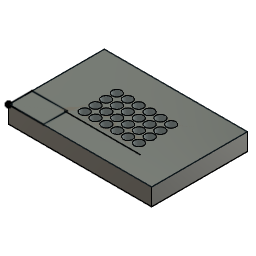
PDT LED Original Array Case Cover v6 (Autodesk Fusion 360 design; units mm, degrees)
Autodesk Fusion 360 part; units mm, degrees
sketch "Sketch1" plane through (0, 0, 0) normal (0, 1, 0) x (1, 0, 0)
  line L0 (0, 0) -> (250, 0)
  line L1 (250, 0) -> (250, -167.253)
  line L2 (250, -167.253) -> (0, -167.253)
  line L3 (0, -167.253) -> (0, 0)
  dimension "d1" = 167.253
  dimension "d2" = 250
  constraint horizontal L0
  constraint vertical L1
  constraint horizontal L2
  constraint vertical L3
  constraint coincident L0.start L3.end
  measures "d1" distance of L0.start L2.end
  measures "d2" distance of L0.start L0.end
extrude "Extrude1" add sketch "Sketch1" along normal blind 30 makes body 1
sketch "Sketch2" plane through (0, 0, 0) normal (0, 1, 0) x (1, 0, 0)
  line L0 (0, 25) -> (127.8, 25)
  line L1 (127.8, 25) -> (127.8, 110.2)
  line L2 (127.8, 110.2) -> (0, 110.2)
  line L3 (0, 110.2) -> (0, 25)
  dimension "d5" = 85.2
  dimension "d6" = 127.8
  constraint horizontal L0
  constraint vertical L1
  constraint horizontal L2
  constraint vertical L3
  measures "d5" distance of L0.start L2.end
  measures "d6" distance of L0.start L0.end
extrude "Extrude2" add sketch "Sketch2" along normal blind 15 separate body makes body 2
sketch "Sketch3" plane through (0, 15, 0) normal (0, 1, 0) x (-1, 0, 0)
  line L0 (0, -110.2) -> (0, -25)
  line L1 (0, -25) -> (-127.8, -25)
  line L2 (-127.8, -25) -> (-127.8, -110.2)
  line L3 (-127.8, -110.2) -> (0, -110.2)
  line L4 (0, -110.2) -> (-16.5, -110.2)
  line L5 (-16.5, -110.2) -> (-16.5, -124.6)
  line L6 (-16.5, -124.6) -> (0, -124.6)
  line L7 (0, -124.6) -> (0, -110.2)
  dimension "d9" = 14.4
  dimension "d10" = 16.5
  constraint horizontal L4
  constraint vertical L5
  constraint horizontal L6
  constraint vertical L7
  constraint coincident L0.start L3.end
  measures "d9" distance of L0.start L6.end
  measures "d10" distance of L0.start L4.end
move_body "Move1" bodies 2 to x (1, 0, 0) y (0, 1, 0) z (0, 0, 1) at (0, 0, -14.638)
hole "Hole1" at (16.5, 15, -110.2) direction (0, -1, 0) diameter 16.3 depth 15 tip angle 118 bodies 2
sketch "Sketch4" plane through (0, 15, 0) normal (0, 1, 0) x (-1, 0, 0)
  circle A0 centre (-16.5, -110.2) radius 8.15
  line L0 (0, -124.838) -> (0, -39.638)
  line L1 (0, -39.638) -> (-127.8, -39.638)
  line L2 (-127.8, -39.638) -> (-127.8, -124.838)
  line L3 (-127.8, -124.838) -> (0, -124.838)
  line L4 (0, -39.638) -> (-16.5, -39.638)
  line L5 (-16.5, -39.638) -> (-16.5, -54.038)
  line L6 (-16.5, -54.038) -> (0, -54.038)
  line L7 (0, -54.038) -> (0, -39.638)
  dimension "d14" = 16.5
  dimension "d15" = 14.4
  constraint horizontal L4
  constraint vertical L5
  constraint horizontal L6
  constraint vertical L7
  constraint coincident L0.end L1.start
  measures "d14" distance of L0.end L4.end
  measures "d15" distance of L0.end L6.end
hole "Hole2" at (16.5, 15, -54.038) direction (0, -1, 0) diameter 16.3 depth 15 tip angle 118 bodies 2
sketch "Sketch5" plane through (0, 15, 0) normal (0, 1, 0) x (-1, 0, 0)
  circle A0 centre (-16.5, -54.038) radius 8.15
  circle A1 centre (-16.5, -110.2) radius 8.15
  line L0 (0, -124.838) -> (0, -39.638)
  line L1 (0, -39.638) -> (-127.8, -39.638)
  line L2 (-127.8, -39.638) -> (-127.8, -124.838)
  line L3 (-127.8, -124.838) -> (0, -124.838)
  line L4 (0, -39.638) -> (-16.5, -39.638)
  line L5 (-16.5, -39.638) -> (-16.5, -72.938)
  line L6 (-16.5, -72.938) -> (0, -72.938)
  line L7 (0, -72.938) -> (0, -39.638)
  dimension "d19" = 33.3
  dimension "d20" = 16.5
  constraint horizontal L4
  constraint vertical L5
  constraint horizontal L6
  constraint vertical L7
  constraint coincident L0.end L1.start
  measures "d19" distance of L0.end L6.end
  measures "d20" distance of L0.end L4.end
hole "Hole3" at (16.5, 15, -72.938) direction (0, -1, 0) diameter 16.3 depth 15 tip angle 118 bodies 2
sketch "Sketch6" plane through (0, 15, 0) normal (0, 1, 0) x (-1, 0, 0)
  circle A0 centre (-16.5, -72.938) radius 8.15
  circle A1 centre (-16.5, -54.038) radius 8.15
  circle A2 centre (-16.5, -110.2) radius 8.15
  line L0 (0, -124.838) -> (0, -39.638)
  line L1 (0, -39.638) -> (-127.8, -39.638)
  line L2 (-127.8, -39.638) -> (-127.8, -124.838)
  line L3 (-127.8, -124.838) -> (0, -124.838)
  line L4 (0, -124.838) -> (-16.5, -124.838)
  line L5 (-16.5, -124.838) -> (-16.5, -91.538)
  line L6 (-16.5, -91.538) -> (0, -91.538)
  line L7 (0, -91.538) -> (0, -124.838)
  dimension "d24" = 33.3
  dimension "d25" = 16.5
  constraint horizontal L4
  constraint vertical L5
  constraint horizontal L6
  constraint vertical L7
  constraint coincident L0.start L3.end
  measures "d24" distance of L0.start L6.end
  measures "d25" distance of L0.start L4.end
hole "Hole4" at (16.5, 15, -91.538) direction (0, -1, 0) diameter 16.3 depth 15 tip angle 118 bodies 2
sketch "Sketch7" plane through (0, 0, -39.638) normal (0, 0, 1) x (1, 0, 0)
  line L0 (0, 0) -> (127.8, 0)
  line L1 (127.8, 0) -> (127.8, 15)
  line L2 (127.8, 15) -> (0, 15)
  line L3 (0, 15) -> (0, 0)
sketch "Sketch8" plane through (0, 15, 0) normal (0, 1, 0) x (-1, 0, 0)
  circle A0 centre (-16.5, -91.538) radius 8.15
  circle A1 centre (-16.5, -72.938) radius 8.15
  circle A2 centre (-16.5, -54.038) radius 8.15
  circle A3 centre (-16.5, -110.2) radius 8.15
  line L0 (0, -124.838) -> (0, -39.638)
  line L1 (0, -39.638) -> (-127.8, -39.638)
  line L2 (-127.8, -39.638) -> (-127.8, -124.838)
  line L3 (-127.8, -124.838) -> (0, -124.838)
  line L4 (0, -39.638) -> (-35.4, -39.638)
  line L5 (-35.4, -39.638) -> (-35.4, -54.038)
  line L6 (-35.4, -54.038) -> (0, -54.038)
  line L7 (0, -54.038) -> (0, -39.638)
  dimension "d29" = 35.4
  dimension "d30" = 14.4
  constraint horizontal L4
  constraint vertical L5
  constraint horizontal L6
  constraint vertical L7
  constraint coincident L0.end L1.start
  measures "d29" distance of L0.end L4.end
  measures "d30" distance of L0.end L6.end
hole "Hole5" at (35.4, 15, -54.038) direction (0, -1, 0) diameter 16.3 depth 15 tip angle 118 bodies 2
sketch "Sketch9" plane through (0, 15, 0) normal (0, 1, 0) x (-1, 0, 0)
  circle A0 centre (-35.4, -54.038) radius 8.15
  circle A1 centre (-16.5, -91.538) radius 8.15
  circle A2 centre (-16.5, -72.938) radius 8.15
  circle A3 centre (-16.5, -54.038) radius 8.15
  circle A4 centre (-16.5, -110.2) radius 8.15
  line L0 (0, -124.838) -> (0, -39.638)
  line L1 (0, -39.638) -> (-127.8, -39.638)
  line L2 (-127.8, -39.638) -> (-127.8, -124.838)
  line L3 (-127.8, -124.838) -> (0, -124.838)
  line L4 (0, -39.638) -> (-35.4, -39.638)
  line L5 (-35.4, -39.638) -> (-35.4, -72.938)
  line L6 (-35.4, -72.938) -> (0, -72.938)
  line L7 (0, -72.938) -> (0, -39.638)
  dimension "d34" = 33.3
  dimension "d35" = 35.4
  constraint horizontal L4
  constraint vertical L5
  constraint horizontal L6
  constraint vertical L7
  constraint coincident L0.end L1.start
  measures "d34" distance of L0.end L6.end
  measures "d35" distance of L0.end L4.end
hole "Hole6" at (35.4, 15, -72.938) direction (0, -1, 0) diameter 16.3 depth 15 tip angle 118 bodies 2
sketch "Sketch10" plane through (0, 15, 0) normal (0, 1, 0) x (-1, 0, 0)
  circle A0 centre (-35.4, -72.938) radius 8.15
  circle A1 centre (-35.4, -54.038) radius 8.15
  circle A2 centre (-16.5, -91.538) radius 8.15
  circle A3 centre (-16.5, -72.938) radius 8.15
  circle A4 centre (-16.5, -54.038) radius 8.15
  circle A5 centre (-16.5, -110.2) radius 8.15
  line L0 (0, -124.838) -> (0, -39.638)
  line L1 (0, -39.638) -> (-127.8, -39.638)
  line L2 (-127.8, -39.638) -> (-127.8, -124.838)
  line L3 (-127.8, -124.838) -> (0, -124.838)
  line L4 (0, -124.838) -> (-35.4, -124.838)
  line L5 (-35.4, -124.838) -> (-35.4, -91.538)
  line L6 (-35.4, -91.538) -> (0, -91.538)
  line L7 (0, -91.538) -> (0, -124.838)
  dimension "d39" = 33.3
  dimension "d40" = 35.4
  constraint horizontal L4
  constraint vertical L5
  constraint horizontal L6
  constraint vertical L7
  constraint coincident L0.start L3.end
  measures "d39" distance of L0.start L6.end
  measures "d40" distance of L0.start L4.end
hole "Hole7" at (35.4, 15, -91.538) direction (0, -1, 0) diameter 16.3 depth 15 tip angle 118 bodies 2
sketch "Sketch11" plane through (0, 15, 0) normal (0, 1, 0) x (-1, 0, 0)
  circle A0 centre (-35.4, -91.538) radius 8.15
  circle A1 centre (-35.4, -72.938) radius 8.15
  circle A2 centre (-35.4, -54.038) radius 8.15
  circle A3 centre (-16.5, -91.538) radius 8.15
  circle A4 centre (-16.5, -72.938) radius 8.15
  circle A5 centre (-16.5, -54.038) radius 8.15
  circle A6 centre (-16.5, -110.2) radius 8.15
  line L0 (0, -124.838) -> (0, -39.638)
  line L1 (0, -39.638) -> (-127.8, -39.638)
  line L2 (-127.8, -39.638) -> (-127.8, -124.838)
  line L3 (-127.8, -124.838) -> (0, -124.838)
  line L4 (0, -124.838) -> (-35.4, -124.838)
  line L5 (-35.4, -124.838) -> (-35.4, -110.438)
  line L6 (-35.4, -110.438) -> (0, -110.438)
  line L7 (0, -110.438) -> (0, -124.838)
  dimension "d44" = 35.4
  dimension "d45" = 14.4
  constraint horizontal L4
  constraint vertical L5
  constraint horizontal L6
  constraint vertical L7
  constraint coincident L0.start L3.end
  measures "d44" distance of L0.start L4.end
  measures "d45" distance of L0.start L6.end
hole "Hole8" at (35.4, 15, -110.438) direction (0, -1, 0) diameter 16.3 depth 15 tip angle 118 bodies 2
sketch "Sketch12" plane through (0, 15, 0) normal (0, 1, 0) x (-1, 0, 0)
  circle A0 centre (-35.4, -110.438) radius 8.15
  circle A1 centre (-35.4, -91.538) radius 8.15
  circle A2 centre (-35.4, -72.938) radius 8.15
  circle A3 centre (-35.4, -54.038) radius 8.15
  circle A4 centre (-16.5, -91.538) radius 8.15
  circle A5 centre (-16.5, -72.938) radius 8.15
  circle A6 centre (-16.5, -54.038) radius 8.15
  circle A7 centre (-16.5, -110.2) radius 8.15
  line L0 (0, -124.838) -> (0, -39.638)
  line L1 (0, -39.638) -> (-127.8, -39.638)
  line L2 (-127.8, -39.638) -> (-127.8, -124.838)
  line L3 (-127.8, -124.838) -> (0, -124.838)
  line L4 (0, -124.838) -> (-54.3, -124.838)
  line L5 (-54.3, -124.838) -> (-54.3, -110.438)
  line L6 (-54.3, -110.438) -> (0, -110.438)
  line L7 (0, -110.438) -> (0, -124.838)
  dimension "d49" = 54.3
  constraint horizontal L4
  constraint vertical L5
  constraint horizontal L6
  constraint vertical L7
  constraint coincident L0.start L3.end
  measures "d49" distance of L0.start L4.end
hole "Hole9" at (54.3, 15, -110.438) direction (0, -1, 0) diameter 16.3 depth 15 tip angle 118 bodies 2
sketch "Sketch13" plane through (0, 15, 0) normal (0, 1, 0) x (-1, 0, 0)
  circle A0 centre (-54.3, -110.438) radius 8.15
  circle A1 centre (-35.4, -110.438) radius 8.15
  circle A2 centre (-35.4, -91.538) radius 8.15
  circle A3 centre (-35.4, -72.938) radius 8.15
  circle A4 centre (-35.4, -54.038) radius 8.15
  circle A5 centre (-16.5, -91.538) radius 8.15
  circle A6 centre (-16.5, -72.938) radius 8.15
  circle A7 centre (-16.5, -54.038) radius 8.15
  circle A8 centre (-16.5, -110.2) radius 8.15
  line L0 (0, -124.838) -> (0, -39.638)
  line L1 (0, -39.638) -> (-127.8, -39.638)
  line L2 (-127.8, -39.638) -> (-127.8, -124.838)
  line L3 (-127.8, -124.838) -> (0, -124.838)
  line L4 (0, -124.838) -> (-54.3, -124.838)
  line L5 (-54.3, -124.838) -> (-54.3, -91.538)
  line L6 (-54.3, -91.538) -> (0, -91.538)
  line L7 (0, -91.538) -> (0, -124.838)
  dimension "d53" = 54.3
  dimension "d54" = 33.3
  constraint horizontal L4
  constraint vertical L5
  constraint horizontal L6
  constraint vertical L7
  constraint coincident L0.start L3.end
  measures "d53" distance of L0.start L4.end
  measures "d54" distance of L0.start L6.end
hole "Hole10" at (54.3, 15, -91.538) direction (0, -1, 0) diameter 16.3 depth 15 tip angle 118 bodies 2
sketch "Sketch14" plane through (0, 15, 0) normal (0, 1, 0) x (-1, 0, 0)
  circle A0 centre (-54.3, -91.538) radius 8.15
  circle A1 centre (-54.3, -110.438) radius 8.15
  circle A2 centre (-35.4, -110.438) radius 8.15
  circle A3 centre (-35.4, -91.538) radius 8.15
  circle A4 centre (-35.4, -72.938) radius 8.15
  circle A5 centre (-35.4, -54.038) radius 8.15
  circle A6 centre (-16.5, -91.538) radius 8.15
  circle A7 centre (-16.5, -72.938) radius 8.15
  circle A8 centre (-16.5, -54.038) radius 8.15
  circle A9 centre (-16.5, -110.2) radius 8.15
  line L0 (0, -124.838) -> (0, -39.638)
  line L1 (0, -39.638) -> (-127.8, -39.638)
  line L2 (-127.8, -39.638) -> (-127.8, -124.838)
  line L3 (-127.8, -124.838) -> (0, -124.838)
  line L4 (0, -39.638) -> (-54.3, -39.638)
  line L5 (-54.3, -39.638) -> (-54.3, -72.938)
  line L6 (-54.3, -72.938) -> (0, -72.938)
  line L7 (0, -72.938) -> (0, -39.638)
  dimension "d58" = 54.3
  dimension "d59" = 33.3
  constraint horizontal L4
  constraint vertical L5
  constraint horizontal L6
  constraint vertical L7
  constraint coincident L0.end L1.start
  measures "d58" distance of L0.end L4.end
  measures "d59" distance of L0.end L6.end
hole "Hole11" at (54.3, 15, -72.938) direction (0, -1, 0) diameter 16.3 depth 15 tip angle 118 bodies 2
sketch "Sketch15" plane through (0, 15, 0) normal (0, 1, 0) x (-1, 0, 0)
  circle A0 centre (-54.3, -72.938) radius 8.15
  circle A1 centre (-54.3, -91.538) radius 8.15
  circle A2 centre (-54.3, -110.438) radius 8.15
  circle A3 centre (-35.4, -110.438) radius 8.15
  circle A4 centre (-35.4, -91.538) radius 8.15
  circle A5 centre (-35.4, -72.938) radius 8.15
  circle A6 centre (-35.4, -54.038) radius 8.15
  circle A7 centre (-16.5, -91.538) radius 8.15
  circle A8 centre (-16.5, -72.938) radius 8.15
  circle A9 centre (-16.5, -54.038) radius 8.15
  circle A10 centre (-16.5, -110.2) radius 8.15
  line L0 (0, -124.838) -> (0, -39.638)
  line L1 (0, -39.638) -> (-127.8, -39.638)
  line L2 (-127.8, -39.638) -> (-127.8, -124.838)
  line L3 (-127.8, -124.838) -> (0, -124.838)
  line L4 (0, -39.638) -> (-54.3, -39.638)
  line L5 (-54.3, -39.638) -> (-54.3, -54.038)
  line L6 (-54.3, -54.038) -> (0, -54.038)
  line L7 (0, -54.038) -> (0, -39.638)
  dimension "d63" = 54.3
  dimension "d64" = 14.4
  constraint horizontal L4
  constraint vertical L5
  constraint horizontal L6
  constraint vertical L7
  constraint coincident L0.end L1.start
  measures "d63" distance of L0.end L4.end
  measures "d64" distance of L0.end L6.end
hole "Hole12" at (54.3, 15, -54.038) direction (0, -1, 0) diameter 16.3 depth 15 tip angle 118 bodies 2
sketch "Sketch16" plane through (0, 15, 0) normal (0, 1, 0) x (-1, 0, 0)
  circle A0 centre (-54.3, -54.038) radius 8.15
  circle A1 centre (-54.3, -72.938) radius 8.15
  circle A2 centre (-54.3, -91.538) radius 8.15
  circle A3 centre (-54.3, -110.438) radius 8.15
  circle A4 centre (-35.4, -110.438) radius 8.15
  circle A5 centre (-35.4, -91.538) radius 8.15
  circle A6 centre (-35.4, -72.938) radius 8.15
  circle A7 centre (-35.4, -54.038) radius 8.15
  circle A8 centre (-16.5, -91.538) radius 8.15
  circle A9 centre (-16.5, -72.938) radius 8.15
  circle A10 centre (-16.5, -54.038) radius 8.15
  circle A11 centre (-16.5, -110.2) radius 8.15
  line L0 (0, -124.838) -> (0, -39.638)
  line L1 (0, -39.638) -> (-127.8, -39.638)
  line L2 (-127.8, -39.638) -> (-127.8, -124.838)
  line L3 (-127.8, -124.838) -> (0, -124.838)
  line L4 (-127.8, -124.838) -> (-73.5, -124.838)
  line L5 (-73.5, -124.838) -> (-73.5, -110.438)
  line L6 (-73.5, -110.438) -> (-127.8, -110.438)
  line L7 (-127.8, -110.438) -> (-127.8, -124.838)
  dimension "d68" = 54.3
  dimension "d69" = 14.4
  constraint horizontal L4
  constraint vertical L5
  constraint horizontal L6
  constraint vertical L7
  constraint coincident L2.end L3.start
  measures "d68" distance of L2.end L4.end
  measures "d69" distance of L2.end L6.end
hole "Hole13" at (73.5, 15, -110.438) direction (0, -1, 0) diameter 16.3 depth 15 tip angle 118 bodies 2
sketch "Sketch17" plane through (0, 15, 0) normal (0, 1, 0) x (-1, 0, 0)
  circle A0 centre (-73.5, -110.438) radius 8.15
  circle A1 centre (-54.3, -54.038) radius 8.15
  circle A2 centre (-54.3, -72.938) radius 8.15
  circle A3 centre (-54.3, -91.538) radius 8.15
  circle A4 centre (-54.3, -110.438) radius 8.15
  circle A5 centre (-35.4, -110.438) radius 8.15
  circle A6 centre (-35.4, -91.538) radius 8.15
  circle A7 centre (-35.4, -72.938) radius 8.15
  circle A8 centre (-35.4, -54.038) radius 8.15
  circle A9 centre (-16.5, -91.538) radius 8.15
  circle A10 centre (-16.5, -72.938) radius 8.15
  circle A11 centre (-16.5, -54.038) radius 8.15
  circle A12 centre (-16.5, -110.2) radius 8.15
  line L0 (0, -124.838) -> (0, -39.638)
  line L1 (0, -39.638) -> (-127.8, -39.638)
  line L2 (-127.8, -39.638) -> (-127.8, -124.838)
  line L3 (-127.8, -124.838) -> (0, -124.838)
  line L4 (-127.8, -124.838) -> (-73.5, -124.838)
  line L5 (-73.5, -124.838) -> (-73.5, -91.538)
  line L6 (-73.5, -91.538) -> (-127.8, -91.538)
  line L7 (-127.8, -91.538) -> (-127.8, -124.838)
  dimension "d73" = 54.3
  dimension "d74" = 33.3
  constraint horizontal L4
  constraint vertical L5
  constraint horizontal L6
  constraint vertical L7
  constraint coincident L2.end L3.start
  measures "d73" distance of L2.end L4.end
  measures "d74" distance of L2.end L6.end
hole "Hole14" at (73.5, 15, -91.538) direction (0, -1, 0) diameter 16.3 depth 15 tip angle 118 bodies 2
sketch "Sketch18" plane through (0, 15, 0) normal (0, 1, 0) x (-1, 0, 0)
  circle A0 centre (-73.5, -91.538) radius 8.15
  circle A1 centre (-73.5, -110.438) radius 8.15
  circle A2 centre (-54.3, -54.038) radius 8.15
  circle A3 centre (-54.3, -72.938) radius 8.15
  circle A4 centre (-54.3, -91.538) radius 8.15
  circle A5 centre (-54.3, -110.438) radius 8.15
  circle A6 centre (-35.4, -110.438) radius 8.15
  circle A7 centre (-35.4, -91.538) radius 8.15
  circle A8 centre (-35.4, -72.938) radius 8.15
  circle A9 centre (-35.4, -54.038) radius 8.15
  circle A10 centre (-16.5, -91.538) radius 8.15
  circle A11 centre (-16.5, -72.938) radius 8.15
  circle A12 centre (-16.5, -54.038) radius 8.15
  circle A13 centre (-16.5, -110.2) radius 8.15
  line L0 (0, -124.838) -> (0, -39.638)
  line L1 (0, -39.638) -> (-127.8, -39.638)
  line L2 (-127.8, -39.638) -> (-127.8, -124.838)
  line L3 (-127.8, -124.838) -> (0, -124.838)
  line L4 (-127.8, -39.638) -> (-73.5, -39.638)
  line L5 (-73.5, -39.638) -> (-73.5, -72.938)
  line L6 (-73.5, -72.938) -> (-127.8, -72.938)
  line L7 (-127.8, -72.938) -> (-127.8, -39.638)
  dimension "d78" = 54.3
  dimension "d79" = 33.3
  constraint horizontal L4
  constraint vertical L5
  constraint horizontal L6
  constraint vertical L7
  constraint coincident L1.end L2.start
  measures "d78" distance of L1.end L4.end
  measures "d79" distance of L1.end L6.end
hole "Hole15" at (73.5, 15, -72.938) direction (0, -1, 0) diameter 16.3 depth 15 tip angle 118 bodies 2
sketch "Sketch19" plane through (0, 15, 0) normal (0, 1, 0) x (-1, 0, 0)
  circle A0 centre (-73.5, -72.938) radius 8.15
  circle A1 centre (-73.5, -91.538) radius 8.15
  circle A2 centre (-73.5, -110.438) radius 8.15
  circle A3 centre (-54.3, -54.038) radius 8.15
  circle A4 centre (-54.3, -72.938) radius 8.15
  circle A5 centre (-54.3, -91.538) radius 8.15
  circle A6 centre (-54.3, -110.438) radius 8.15
  circle A7 centre (-35.4, -110.438) radius 8.15
  circle A8 centre (-35.4, -91.538) radius 8.15
  circle A9 centre (-35.4, -72.938) radius 8.15
  circle A10 centre (-35.4, -54.038) radius 8.15
  circle A11 centre (-16.5, -91.538) radius 8.15
  circle A12 centre (-16.5, -72.938) radius 8.15
  circle A13 centre (-16.5, -54.038) radius 8.15
  circle A14 centre (-16.5, -110.2) radius 8.15
  line L0 (0, -124.838) -> (0, -39.638)
  line L1 (0, -39.638) -> (-127.8, -39.638)
  line L2 (-127.8, -39.638) -> (-127.8, -124.838)
  line L3 (-127.8, -124.838) -> (0, -124.838)
  line L4 (-127.8, -39.638) -> (-73.5, -39.638)
  line L5 (-73.5, -39.638) -> (-73.5, -54.038)
  line L6 (-73.5, -54.038) -> (-127.8, -54.038)
  line L7 (-127.8, -54.038) -> (-127.8, -39.638)
  dimension "d83" = 54.3
  dimension "d84" = 14.4
  constraint horizontal L4
  constraint vertical L5
  constraint horizontal L6
  constraint vertical L7
  constraint coincident L1.end L2.start
  measures "d83" distance of L1.end L4.end
  measures "d84" distance of L1.end L6.end
hole "Hole16" at (73.5, 15, -54.038) direction (0, -1, 0) diameter 16.3 depth 15 tip angle 118 bodies 2
sketch "Sketch20" plane through (0, 15, 0) normal (0, 1, 0) x (-1, 0, 0)
  circle A0 centre (-73.5, -54.038) radius 8.15
  circle A1 centre (-73.5, -72.938) radius 8.15
  circle A2 centre (-73.5, -91.538) radius 8.15
  circle A3 centre (-73.5, -110.438) radius 8.15
  circle A4 centre (-54.3, -54.038) radius 8.15
  circle A5 centre (-54.3, -72.938) radius 8.15
  circle A6 centre (-54.3, -91.538) radius 8.15
  circle A7 centre (-54.3, -110.438) radius 8.15
  circle A8 centre (-35.4, -110.438) radius 8.15
  circle A9 centre (-35.4, -91.538) radius 8.15
  circle A10 centre (-35.4, -72.938) radius 8.15
  circle A11 centre (-35.4, -54.038) radius 8.15
  circle A12 centre (-16.5, -91.538) radius 8.15
  circle A13 centre (-16.5, -72.938) radius 8.15
  circle A14 centre (-16.5, -54.038) radius 8.15
  circle A15 centre (-16.5, -110.2) radius 8.15
  line L0 (0, -124.838) -> (0, -39.638)
  line L1 (0, -39.638) -> (-127.8, -39.638)
  line L2 (-127.8, -39.638) -> (-127.8, -124.838)
  line L3 (-127.8, -124.838) -> (0, -124.838)
  line L4 (-127.8, -39.638) -> (-92.4, -39.638)
  line L5 (-92.4, -39.638) -> (-92.4, -54.038)
  line L6 (-92.4, -54.038) -> (-127.8, -54.038)
  line L7 (-127.8, -54.038) -> (-127.8, -39.638)
  dimension "d88" = 35.4
  constraint horizontal L4
  constraint vertical L5
  constraint horizontal L6
  constraint vertical L7
  constraint coincident L1.end L2.start
  measures "d88" distance of L1.end L4.end
hole "Hole17" at (92.4, 15, -54.038) direction (0, -1, 0) diameter 16.3 depth 15 tip angle 118 bodies 2
sketch "Sketch21" plane through (0, 15, 0) normal (0, 1, 0) x (-1, 0, 0)
  circle A0 centre (-92.4, -54.038) radius 8.15
  circle A1 centre (-73.5, -54.038) radius 8.15
  circle A2 centre (-73.5, -72.938) radius 8.15
  circle A3 centre (-73.5, -91.538) radius 8.15
  circle A4 centre (-73.5, -110.438) radius 8.15
  circle A5 centre (-54.3, -54.038) radius 8.15
  circle A6 centre (-54.3, -72.938) radius 8.15
  circle A7 centre (-54.3, -91.538) radius 8.15
  circle A8 centre (-54.3, -110.438) radius 8.15
  circle A9 centre (-35.4, -110.438) radius 8.15
  circle A10 centre (-35.4, -91.538) radius 8.15
  circle A11 centre (-35.4, -72.938) radius 8.15
  circle A12 centre (-35.4, -54.038) radius 8.15
  circle A13 centre (-16.5, -91.538) radius 8.15
  circle A14 centre (-16.5, -72.938) radius 8.15
  circle A15 centre (-16.5, -54.038) radius 8.15
  circle A16 centre (-16.5, -110.2) radius 8.15
  line L0 (0, -124.838) -> (0, -39.638)
  line L1 (0, -39.638) -> (-127.8, -39.638)
  line L2 (-127.8, -39.638) -> (-127.8, -124.838)
  line L3 (-127.8, -124.838) -> (0, -124.838)
  line L4 (-127.8, -39.638) -> (-92.4, -39.638)
  line L5 (-92.4, -39.638) -> (-92.4, -72.938)
  line L6 (-92.4, -72.938) -> (-127.8, -72.938)
  line L7 (-127.8, -72.938) -> (-127.8, -39.638)
  dimension "d92" = 33.3
  dimension "d93" = 35.4
  constraint horizontal L4
  constraint vertical L5
  constraint horizontal L6
  constraint vertical L7
  constraint coincident L1.end L2.start
  measures "d92" distance of L1.end L6.end
  measures "d93" distance of L1.end L4.end
hole "Hole18" at (92.4, 15, -72.938) direction (0, -1, 0) diameter 16.3 depth 15 tip angle 118 bodies 2
sketch "Sketch22" plane through (0, 15, 0) normal (0, 1, 0) x (-1, 0, 0)
  circle A0 centre (-92.4, -72.938) radius 8.15
  circle A1 centre (-92.4, -54.038) radius 8.15
  circle A2 centre (-73.5, -54.038) radius 8.15
  circle A3 centre (-73.5, -72.938) radius 8.15
  circle A4 centre (-73.5, -91.538) radius 8.15
  circle A5 centre (-73.5, -110.438) radius 8.15
  circle A6 centre (-54.3, -54.038) radius 8.15
  circle A7 centre (-54.3, -72.938) radius 8.15
  circle A8 centre (-54.3, -91.538) radius 8.15
  circle A9 centre (-54.3, -110.438) radius 8.15
  circle A10 centre (-35.4, -110.438) radius 8.15
  circle A11 centre (-35.4, -91.538) radius 8.15
  circle A12 centre (-35.4, -72.938) radius 8.15
  circle A13 centre (-35.4, -54.038) radius 8.15
  circle A14 centre (-16.5, -91.538) radius 8.15
  circle A15 centre (-16.5, -72.938) radius 8.15
  circle A16 centre (-16.5, -54.038) radius 8.15
  circle A17 centre (-16.5, -110.2) radius 8.15
  line L0 (0, -124.838) -> (0, -39.638)
  line L1 (0, -39.638) -> (-127.8, -39.638)
  line L2 (-127.8, -39.638) -> (-127.8, -124.838)
  line L3 (-127.8, -124.838) -> (0, -124.838)
  line L4 (-127.8, -124.838) -> (-92.4, -124.838)
  line L5 (-92.4, -124.838) -> (-92.4, -91.538)
  line L6 (-92.4, -91.538) -> (-127.8, -91.538)
  line L7 (-127.8, -91.538) -> (-127.8, -124.838)
  dimension "d97" = 35.4
  dimension "d98" = 33.3
  constraint horizontal L4
  constraint vertical L5
  constraint horizontal L6
  constraint vertical L7
  constraint coincident L2.end L3.start
  measures "d97" distance of L2.end L4.end
  measures "d98" distance of L2.end L6.end
hole "Hole19" at (92.4, 15, -91.538) direction (0, -1, 0) diameter 16.3 depth 15 tip angle 118 bodies 2
sketch "Sketch23" plane through (0, 15, 0) normal (0, 1, 0) x (-1, 0, 0)
  circle A0 centre (-92.4, -91.538) radius 8.15
  circle A1 centre (-92.4, -72.938) radius 8.15
  circle A2 centre (-92.4, -54.038) radius 8.15
  circle A3 centre (-73.5, -54.038) radius 8.15
  circle A4 centre (-73.5, -72.938) radius 8.15
  circle A5 centre (-73.5, -91.538) radius 8.15
  circle A6 centre (-73.5, -110.438) radius 8.15
  circle A7 centre (-54.3, -54.038) radius 8.15
  circle A8 centre (-54.3, -72.938) radius 8.15
  circle A9 centre (-54.3, -91.538) radius 8.15
  circle A10 centre (-54.3, -110.438) radius 8.15
  circle A11 centre (-35.4, -110.438) radius 8.15
  circle A12 centre (-35.4, -91.538) radius 8.15
  circle A13 centre (-35.4, -72.938) radius 8.15
  circle A14 centre (-35.4, -54.038) radius 8.15
  circle A15 centre (-16.5, -91.538) radius 8.15
  circle A16 centre (-16.5, -72.938) radius 8.15
  circle A17 centre (-16.5, -54.038) radius 8.15
  circle A18 centre (-16.5, -110.2) radius 8.15
  line L0 (0, -124.838) -> (0, -39.638)
  line L1 (0, -39.638) -> (-127.8, -39.638)
  line L2 (-127.8, -39.638) -> (-127.8, -124.838)
  line L3 (-127.8, -124.838) -> (0, -124.838)
  line L4 (-127.8, -124.838) -> (-92.4, -124.838)
  line L5 (-92.4, -124.838) -> (-92.4, -110.438)
  line L6 (-92.4, -110.438) -> (-127.8, -110.438)
  line L7 (-127.8, -110.438) -> (-127.8, -124.838)
  dimension "d102" = 35.4
  dimension "d103" = 14.4
  constraint horizontal L4
  constraint vertical L5
  constraint horizontal L6
  constraint vertical L7
  constraint coincident L2.end L3.start
  measures "d102" distance of L2.end L4.end
  measures "d103" distance of L2.end L6.end
hole "Hole20" at (92.4, 15, -110.438) direction (0, -1, 0) diameter 16.3 depth 15 tip angle 118 bodies 2
sketch "Sketch24" plane through (0, 15, 0) normal (0, 1, 0) x (-1, 0, 0)
  circle A0 centre (-92.4, -110.438) radius 8.15
  circle A1 centre (-92.4, -91.538) radius 8.15
  circle A2 centre (-92.4, -72.938) radius 8.15
  circle A3 centre (-92.4, -54.038) radius 8.15
  circle A4 centre (-73.5, -54.038) radius 8.15
  circle A5 centre (-73.5, -72.938) radius 8.15
  circle A6 centre (-73.5, -91.538) radius 8.15
  circle A7 centre (-73.5, -110.438) radius 8.15
  circle A8 centre (-54.3, -54.038) radius 8.15
  circle A9 centre (-54.3, -72.938) radius 8.15
  circle A10 centre (-54.3, -91.538) radius 8.15
  circle A11 centre (-54.3, -110.438) radius 8.15
  circle A12 centre (-35.4, -110.438) radius 8.15
  circle A13 centre (-35.4, -91.538) radius 8.15
  circle A14 centre (-35.4, -72.938) radius 8.15
  circle A15 centre (-35.4, -54.038) radius 8.15
  circle A16 centre (-16.5, -91.538) radius 8.15
  circle A17 centre (-16.5, -72.938) radius 8.15
  circle A18 centre (-16.5, -54.038) radius 8.15
  circle A19 centre (-16.5, -110.2) radius 8.15
  line L0 (0, -124.838) -> (0, -39.638)
  line L1 (0, -39.638) -> (-127.8, -39.638)
  line L2 (-127.8, -39.638) -> (-127.8, -124.838)
  line L3 (-127.8, -124.838) -> (0, -124.838)
  line L4 (-127.8, -124.838) -> (-111.3, -124.838)
  line L5 (-111.3, -124.838) -> (-111.3, -110.438)
  line L6 (-111.3, -110.438) -> (-127.8, -110.438)
  line L7 (-127.8, -110.438) -> (-127.8, -124.838)
  dimension "d107" = 16.5
  dimension "d108" = 14.4
  constraint horizontal L4
  constraint vertical L5
  constraint horizontal L6
  constraint vertical L7
  constraint coincident L2.end L3.start
  measures "d107" distance of L2.end L4.end
  measures "d108" distance of L2.end L6.end
hole "Hole21" at (111.3, 15, -110.438) direction (0, -1, 0) diameter 16.3 depth 15 tip angle 118 bodies 2
sketch "Sketch25" plane through (0, 15, 0) normal (0, 1, 0) x (-1, 0, 0)
  circle A0 centre (-111.3, -110.438) radius 8.15
  circle A1 centre (-92.4, -110.438) radius 8.15
  circle A2 centre (-92.4, -91.538) radius 8.15
  circle A3 centre (-92.4, -72.938) radius 8.15
  circle A4 centre (-92.4, -54.038) radius 8.15
  circle A5 centre (-73.5, -54.038) radius 8.15
  circle A6 centre (-73.5, -72.938) radius 8.15
  circle A7 centre (-73.5, -91.538) radius 8.15
  circle A8 centre (-73.5, -110.438) radius 8.15
  circle A9 centre (-54.3, -54.038) radius 8.15
  circle A10 centre (-54.3, -72.938) radius 8.15
  circle A11 centre (-54.3, -91.538) radius 8.15
  circle A12 centre (-54.3, -110.438) radius 8.15
  circle A13 centre (-35.4, -110.438) radius 8.15
  circle A14 centre (-35.4, -91.538) radius 8.15
  circle A15 centre (-35.4, -72.938) radius 8.15
  circle A16 centre (-35.4, -54.038) radius 8.15
  circle A17 centre (-16.5, -91.538) radius 8.15
  circle A18 centre (-16.5, -72.938) radius 8.15
  circle A19 centre (-16.5, -54.038) radius 8.15
  circle A20 centre (-16.5, -110.2) radius 8.15
  line L0 (0, -124.838) -> (0, -39.638)
  line L1 (0, -39.638) -> (-127.8, -39.638)
  line L2 (-127.8, -39.638) -> (-127.8, -124.838)
  line L3 (-127.8, -124.838) -> (0, -124.838)
  line L4 (-127.8, -124.838) -> (-111.3, -124.838)
  line L5 (-111.3, -124.838) -> (-111.3, -91.538)
  line L6 (-111.3, -91.538) -> (-127.8, -91.538)
  line L7 (-127.8, -91.538) -> (-127.8, -124.838)
  dimension "d112" = 33.3
  dimension "d113" = 16.5
  constraint horizontal L4
  constraint vertical L5
  constraint horizontal L6
  constraint vertical L7
  constraint coincident L2.end L3.start
  measures "d112" distance of L2.end L6.end
  measures "d113" distance of L2.end L4.end
hole "Hole22" at (111.3, 15, -91.538) direction (0, -1, 0) diameter 16.3 depth 15 tip angle 118 bodies 2
sketch "Sketch26" plane through (0, 0, 0) normal (0, -1, 0) x (1, 0, 0)
  circle A0 centre (111.3, -91.538) radius 8.15
  circle A1 centre (111.3, -110.438) radius 8.15
  circle A2 centre (92.4, -110.438) radius 8.15
  circle A3 centre (92.4, -91.538) radius 8.15
  circle A4 centre (92.4, -72.938) radius 8.15
  circle A5 centre (92.4, -54.038) radius 8.15
  circle A6 centre (73.5, -54.038) radius 8.15
  circle A7 centre (73.5, -72.938) radius 8.15
  circle A8 centre (73.5, -91.538) radius 8.15
  circle A9 centre (73.5, -110.438) radius 8.15
  circle A10 centre (54.3, -54.038) radius 8.15
  circle A11 centre (54.3, -72.938) radius 8.15
  circle A12 centre (54.3, -91.538) radius 8.15
  circle A13 centre (54.3, -110.438) radius 8.15
  circle A14 centre (35.4, -110.438) radius 8.15
  circle A15 centre (35.4, -91.538) radius 8.15
  circle A16 centre (35.4, -72.938) radius 8.15
  circle A17 centre (35.4, -54.038) radius 8.15
  circle A18 centre (16.5, -91.538) radius 8.15
  circle A19 centre (16.5, -72.938) radius 8.15
  circle A20 centre (16.5, -54.038) radius 8.15
  circle A21 centre (16.5, -110.2) radius 8.15
  line L0 (0, -39.638) -> (0, -124.838)
  line L1 (0, -124.838) -> (127.8, -124.838)
  line L2 (127.8, -124.838) -> (127.8, -39.638)
  line L3 (127.8, -39.638) -> (0, -39.638)
  line L4 (127.8, -39.638) -> (111.3, -39.638)
  line L5 (111.3, -39.638) -> (111.3, -72.938)
  line L6 (111.3, -72.938) -> (127.8, -72.938)
  line L7 (127.8, -72.938) -> (127.8, -39.638)
  dimension "d117" = 33.3
  dimension "d118" = 16.5
  constraint horizontal L4
  constraint vertical L5
  constraint horizontal L6
  constraint vertical L7
  constraint coincident L2.end L3.start
  measures "d117" distance of L2.end L6.end
  measures "d118" distance of L2.end L4.end
hole "Hole23" at (111.3, 0, -72.938) direction (0, 1, 0) diameter 16.3 depth 15 tip angle 118 bodies 2
sketch "Sketch27" plane through (0, 15, 0) normal (0, 1, 0) x (-1, 0, 0)
  circle A0 centre (-111.3, -72.938) radius 8.15
  circle A1 centre (-111.3, -91.538) radius 8.15
  circle A2 centre (-111.3, -110.438) radius 8.15
  circle A3 centre (-92.4, -110.438) radius 8.15
  circle A4 centre (-92.4, -91.538) radius 8.15
  circle A5 centre (-92.4, -72.938) radius 8.15
  circle A6 centre (-92.4, -54.038) radius 8.15
  circle A7 centre (-73.5, -54.038) radius 8.15
  circle A8 centre (-73.5, -72.938) radius 8.15
  circle A9 centre (-73.5, -91.538) radius 8.15
  circle A10 centre (-73.5, -110.438) radius 8.15
  circle A11 centre (-54.3, -54.038) radius 8.15
  circle A12 centre (-54.3, -72.938) radius 8.15
  circle A13 centre (-54.3, -91.538) radius 8.15
  circle A14 centre (-54.3, -110.438) radius 8.15
  circle A15 centre (-35.4, -110.438) radius 8.15
  circle A16 centre (-35.4, -91.538) radius 8.15
  circle A17 centre (-35.4, -72.938) radius 8.15
  circle A18 centre (-35.4, -54.038) radius 8.15
  circle A19 centre (-16.5, -91.538) radius 8.15
  circle A20 centre (-16.5, -72.938) radius 8.15
  circle A21 centre (-16.5, -54.038) radius 8.15
  circle A22 centre (-16.5, -110.2) radius 8.15
  line L0 (0, -124.838) -> (0, -39.638)
  line L1 (0, -39.638) -> (-127.8, -39.638)
  line L2 (-127.8, -39.638) -> (-127.8, -124.838)
  line L3 (-127.8, -124.838) -> (0, -124.838)
  line L4 (-127.8, -39.638) -> (-111.3, -39.638)
  line L5 (-111.3, -39.638) -> (-111.3, -54.038)
  line L6 (-111.3, -54.038) -> (-127.8, -54.038)
  line L7 (-127.8, -54.038) -> (-127.8, -39.638)
  dimension "d122" = 16.5
  dimension "d123" = 14.4
  constraint horizontal L4
  constraint vertical L5
  constraint horizontal L6
  constraint vertical L7
  constraint coincident L1.end L2.start
  measures "d122" distance of L1.end L4.end
  measures "d123" distance of L1.end L6.end
hole "Hole24" at (111.3, 15, -54.038) direction (0, -1, 0) diameter 16.3 depth 15 tip angle 118 bodies 2
sketch "Sketch28" plane through (0, 30, 0) normal (0, 1, 0) x (-1, 0, 0)
  line L0 (0, 167.253) -> (-250, 167.253)
  line L1 (-250, 167.253) -> (-250, 0)
  line L2 (-250, 0) -> (0, 0)
  line L3 (0, 0) -> (0, 167.253)
  line L4 (0, 167.253) -> (-61.1, 167.253)
  line L5 (-61.1, 167.253) -> (-61.1, 126.3765)
  line L6 (-61.1, 126.3765) -> (0, 126.3765)
  line L7 (0, 126.3765) -> (0, 167.253)
  dimension "d127" = 40.8765
  dimension "d128" = 61.1
  constraint horizontal L4
  constraint vertical L5
  constraint horizontal L6
  constraint vertical L7
  constraint coincident L0.start L3.end
  measures "d127" distance of L0.start L6.end
  measures "d128" distance of L0.start L4.end
sketch "Sketch29" plane through (0, 30, 0) normal (0, 1, 0) x (-1, 0, 0)
  line L0 (-61, 126.5) -> (-188.8, 126.5)
  line L1 (-188.8, 126.5) -> (-188.8, 41)
  line L2 (-188.8, 41) -> (-61, 41)
  line L3 (-61, 41) -> (-61, 126.5)
  dimension "d129" = 127.8
  dimension "d130" = 85.5
  constraint horizontal L0
  constraint vertical L1
  constraint horizontal L2
  constraint vertical L3
  measures "d129" distance of L0.start L0.end
  measures "d130" distance of L0.start L2.end
extrude "Extrude3" cut sketch "Sketch29" against normal blind 30 bodies 1
extrude "Extrude4" cut 1 faces at (103.6, 20, 126.5) along direction (0, 0, 1) blind 2 on bodies 1 bodies 1
extrude "Extrude5" cut 1 faces at (188.8, 10, 99.3333) along direction (1, 0, 0) blind 2 on bodies 1 bodies 1
extrude "Extrude6" cut 1 faces at (147.5333, 20, 41) along direction (0, 0, -1) blind 2 on bodies 1 bodies 1
extrude "Extrude7" cut 1 faces at (61, 10, 68.8333) along direction (-1, 0, 0) blind 2 on bodies 1 bodies 1
extrude "Extrude8" add 1 faces at (127.8, 10, -68.038) along direction (1, 0, 0) blind 2 on bodies 2 bodies 2
extrude "Extrude9" add sketch "Sketch7" along normal blind 2 bodies 2
extrude "Extrude10" add 1 faces at (127.8, 5, -38.9713) along direction (1, 0, 0) blind 2 on bodies 2 bodies 2
extrude "Extrude11" add 1 faces at (86.5333, 10, -124.838) along direction (0, 0, -1) blind 2 on bodies 2 bodies 2
extrude "Extrude12" add 1 faces at (0, 10, -97.1046) along direction (-1, 0, 0) blind 2 on bodies 2 bodies 2
move_body "Move2" bodies 2 to x (1, 0, 0) y (0, 1, 0) z (0, 0, 1) at (61.3389, -38.8162, 166.2396)
move_body "Move3" bodies 2 to x (1, 0, 0) y (0, 1, 0) z (0, 0, 1) at (6.2919, 0, 6.2919)
move_body "Move4" bodies 2 to x (1, 0, 0) y (0, 1, 0) z (0, 0, 1) at (-6.6308, 53.8162, -6.6936)
combine "Combine1" operation add target body 2 tool bodies 1
